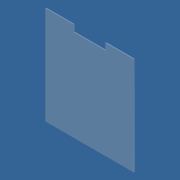
# Autodesk Inventor part: top plate
Saved by Autodesk Inventor 2012 (Build 160160000, 160)
## iProperties
Created: 2012-03-16
Part Number: top plate
Material: Polycarbonate, Clear
Document SubType Name: Modeling
Designer: Ed
Mass: 1937.93 g
Surface Area: 5215.15 cm^2
Volume: 1614.95 cm^3
Density: 1.2 g/cm^3
Author: Ed
Autodesk Inventor part; units mm, degrees
ref_plane "YZ Plane" through (0, 0, 0) normal (1, 0, 0) x (0, 1, 0)
ref_plane "XZ Plane" through (0, 0, 0) normal (0, 1, 0) x (-1, 0, 0)
ref_plane "XY Plane" through (0, 0, 0) normal (0, 0, 1) x (1, 0, 0)
sketch "Sketch1" plane through (0, 0, 0) normal (0, 0, 1) x (1, 0, 0)
  line L0 (0, 0) -> (530.86, 0)
  line L1 (530.86, 0) -> (530.86, 589.28)
  line L2 (530.86, 589.28) -> (0, 589.28)
  line L3 (0, 589.28) -> (0, 0)
  line L4 (170.18, 589.28) -> (360.68, 589.28)
  line L5 (360.68, 589.28) -> (360.68, 549.28)
  line L6 (360.68, 549.28) -> (170.18, 549.28)
  line L7 (170.18, 549.28) -> (170.18, 589.28)
  point P0 (265.43, 589.28)
  dimension "d0" = 589.28
  dimension "d1" = 530.86
  dimension "d4" = 40
  dimension "d5" = 190.5
  constraints: 16 end point, 4 parallel, 2 horizontal, 2 midpoint, 2 perpendicular, 1 point on line
  measures "d0" distance of L2.end L0.start
  measures "d1" distance of L0.start L0.end
  measures "d4" distance of L4.end L5.end
  measures "d5" distance of L5.end L6.end
extrude "Extrusion1" add sketch "Sketch1" along normal blind 6.35 contours L3 L2 L7 L6 L5 L1 L0
body "Solid1"
